Autodesk Fusion 360 part; units mm, degrees
(part 6 of 6)
sketch "Button Layout" plane through (0, 0, 6) normal (0, 0, 1) x (-1, 0, 0)
  line L0 (0, -86.085) -> (0, 0)
  line L1 (0, 0) -> (-270, 0)
  line L2 (-270, 0) -> (-270, -86.085)
  line L3 (-270, -86.085) -> (0, -86.085)
  circle A0 centre (-90, -43) radius 15
  circle A1 centre (-140, -43) radius 15
  circle A2 centre (-40, -43) radius 15
  dimension "d12" = 30
  dimension "d13" = 30
  dimension "d14" = 30
  dimension "d17" = 40
  dimension "d20" = 50
  dimension "d21" = 43
  dimension "d22" = 43
  dimension "d23" = 43
  dimension "d24" = 50
  measures "d12" diameter of A0
  measures "d13" diameter of A1
  measures "d14" diameter of A2
  measures "d17" distance of L0 A2.centre
  measures "d20" distance of A0.centre A1.centre
  measures "d21" distance of L1 A2.centre
  measures "d22" distance of L1 A0.centre
  measures "d23" distance of L1 A1.centre
  measures "d24" distance of A0.centre A2.centre
extrude "Extrude2" cut sketch "Button Layout" against normal blind 6 contours A0 | A1
extrude "Extrude3" cut sketch "Button Layout" against normal blind 6 contours A2
equation "MDFThickness = 6 mm"
equation "d2 = MDFThickness"
equation "controlPanelTopLength = 75 mm"
equation "controlPanelTopWidth = 250 mm"
equation "arcadeButtonDiameter = 30 mm"
equation "d12 = arcadeButtonDiameter"
equation "d13 = arcadeButtonDiameter"
equation "d14 = arcadeButtonDiameter"
equation "d21 = ( 86 / 2 ) * 1 mm"
equation "d22 = ( 86 / 2 ) * 1 mm"
equation "d23 = ( 86 / 2 ) * 1 mm"

design "Sorted Smarties Cover Connector Base"
Autodesk Fusion 360 part; units mm, degrees
sketch "Sorted Smarties Cover Connector Base" plane through (0, 0, 0) normal (0, 0, 1) x (1, 0, 0)
  line L0 (0, 0) -> (30, 0)
  line L1 (30, 0) -> (30, 15)
  line L2 (30, 15) -> (0, 15)
  line L3 (0, 15) -> (0, 0)
  dimension "d5" = 15
  dimension "d6" = 30
  constraint horizontal L0
  constraint vertical L1
  constraint horizontal L2
  constraint vertical L3
  constraint coincident L0.start L3.end
  measures "d5" distance of L0.start L2.end
  measures "d6" distance of L0.start L0.end
extrude "Extrude1" add sketch "Sorted Smarties Cover Connector Base" along normal blind 15
sketch "Connecting Section" plane through (0, 0, 15) normal (0, 0, 1) x (-1, 0, 0)
  line L0 (0, -15) -> (0, 0)
  line L1 (0, 0) -> (-30, 0)
  line L2 (-30, 0) -> (-30, -15)
  line L3 (-30, -15) -> (0, -15)
  line L4 (-30, -11) -> (-4, -11)
  line L5 (-4, -11) -> (-4, -4)
  line L6 (-4, -4) -> (-30, -4)
  line L7 (-30, -4) -> (-30, -11)
  dimension "d7" = 7
  dimension "d8" = 4
  dimension "d9" = 4
  dimension "d10" = 4
  constraint horizontal L4
  constraint vertical L5
  constraint horizontal L6
  constraint vertical L7
  constraint coincident L2 L4.start
  measures "d7" distance of L4 L6
  measures "d8" distance of L1 L6
  measures "d9" distance of L3 L4
  measures "d10" distance of L0 L5
extrude "Extrude2" cut sketch "Connecting Section" against normal blind 11 contours L2 L4 L5 L6 L7
equation "d8 = ( ( 15 - 7 ) / 2 ) * 1 mm"

design "Top Panel"
Autodesk Fusion 360 part; units mm, degrees
sketch "Top Panel" plane through (0, 0, 0) normal (1, 0, 0) x (0, 1, 0)
  line L0 (-0.0158, 146.1836) -> (175.2958, 74.2831)
  line L1 (175.2958, 80.7681) -> (-0.0158, 152.6686)
  line L2 (-0.0158, 152.6686) -> (-0.0158, 146.1836)
  line L3 (175.2958, 80.7681) -> (175.2958, 74.2831)
  dimension "d12" = 189.483
  dimension "d13" = 189.483
  dimension "d14" = 6
  dimension "d18" = 67.7
  constraint vertical L2
  constraint parallel L2 L3
  measures "d12" distance of L1.start L1.end
  measures "d13" distance of L0.start L0.end
  measures "d14" distance of L0 L1
  measures "d18" angle of L0 L3
extrude "Extrude2" add sketch "Top Panel" along normal blind 270
equation "MDFThickness = 6 mm"
equation "topPlateWidth = 210 mm"
equation "baseBreadth = 250 mm"
equation "filletRadius = 8 mm"

design "Lower Wire Management Conduit"
Autodesk Fusion 360 part; units mm, degrees
sketch "16 mm x 16 mm conduit piping shape" plane through (0, 0, 0) normal (1, 0, 0) x (0, 1, 0)
  line L0 (0, 0) -> (16, 0)
  line L1 (16, 0) -> (16, 10)
  line L2 (16, 10) -> (14, 13.9)
  line L3 (14, 13.9) -> (13.1102, 13.4437)
  line L4 (13.1102, 13.4437) -> (15, 9.7585)
  line L5 (15, 9.7585) -> (15, 1)
  line L6 (15, 1) -> (1, 1)
  line L7 (1, 1) -> (1, 9.7585)
  line L8 (1, 9.7585) -> (2.8898, 13.4437)
  line L9 (2.8898, 13.4437) -> (2, 13.9)
  line L10 (2, 13.9) -> (0, 10)
  line L11 (0, 10) -> (0, 0)
  line L12 (0, 16) -> (16, 16)
  line L13 (0, 16) -> (0, 12)
  line L14 (0, 12) -> (1, 12)
  line L15 (1, 12) -> (1, 15)
  line L16 (1, 15) -> (15, 15)
  line L17 (15, 15) -> (15, 12)
  line L18 (15, 12) -> (16, 12)
  line L19 (16, 12) -> (16, 16)
  dimension "d1" = 1
  dimension "d2" = 16
  dimension "d3" = 1
  dimension "d4" = 1
  dimension "d7" = 10
  dimension "d8" = 10
  dimension "d9" = 16
  dimension "d10" = 1
  dimension "d11" = 1
  dimension "d12" = 1
  dimension "d13" = 4
  dimension "d14" = 4
  dimension "d15" = 16
  dimension "d16" = 2
  dimension "d17" = 2
  dimension "d18" = 1
  dimension "d19" = 1
  constraint coincident L0.start L11.end
  constraint horizontal L0
  constraint perpendicular L0 L1
  constraint perpendicular L2 L3
  constraint parallel L1 L5
  constraint perpendicular L5 L6
  constraint perpendicular L6 L7
  constraint perpendicular L0 L11
  constraint horizontal L12
  constraint perpendicular L12 L13
  constraint perpendicular L13 L14
  constraint perpendicular L14 L15
  constraint perpendicular L15 L16
  constraint perpendicular L16 L17
  constraint perpendicular L17 L18
  constraint perpendicular L12 L19
  constraint parallel L8 L10
  constraint parallel L2 L4
  constraint perpendicular L9 L10
  measures "d1" distance of L0 L6
  measures "d2" distance of L1 L11
  measures "d3" distance of L7 L11
  measures "d4" distance of L1 L5
  measures "d7" distance of L0.end L1.end
  measures "d8" distance of L10.end L0.start
  measures "d9" distance of L0 L12
  measures "d10" distance of L12 L16
  measures "d11" distance of L17 L19
  measures "d12" distance of L13 L15
  measures "d13" distance of L12.end L18.end
  measures "d14" distance of L12.start L13.end
  measures "d15" distance of L12.start L12.end
  measures "d16" distance of L1.end L2.end
  measures "d17" distance of L9.end L10.end
  measures "d18" distance of L2.end L3.end
  measures "d19" distance of L8.end L9.end
extrude "Extrude1" add sketch "16 mm x 16 mm conduit piping shape" along normal blind 182 makes body 1 at (60.6667, 5.3333, 16) makes body 2 at (60.6667, 5.3333, 0)
fillet "Fillet1" radius 0.3 18 edges at (91, 0, 16) (91, 16, 16) (91, 16, 12) (91, 0, 12) (91, 1, 12) (91, 15, 12) (91, 1, 15) (91, 15, 15) (91, 0, 10) (91, 16, 10) (91, 14, 13.9) (91, 13.1102, 13.4437) (91, 2, 13.9) (91, 2.8898, 13.4437) (91, 15, 1) (91, 1, 1) (91, 1, 9.7585) (91, 15, 9.7585) on bodies 1 2
equation "d1 = conduitThickness"
equation "d2 = conduitWidth"
equation "d3 = conduitThickness"
equation "d4 = conduitThickness"
equation "conduitThickness = 1 mm"
equation "conduitWidth = 16 mm"
equation "d9 = conduitWidth"
equation "d10 = conduitThickness"
equation "d11 = conduitThickness"
equation "d12 = conduitThickness"
equation "d20 = ( 234 mm ) - ( 2 * ( 26 ) ) * 1 mm"

design "Sorted Smarties Top Support Right"
Autodesk Fusion 360 part; units mm, degrees
sketch "Back Panel Support Left " plane through (0, 0, 0) normal (1, 0, 0) x (0, 1, 0)
  line L0 (0, 0) -> (28, 0)
  line L1 (28, 0) -> (28, 21)
  line L2 (28, 21) -> (0, 21)
  line L3 (0, 21) -> (0, 0)
  dimension "d1" = 21
  dimension "d2" = 28
  constraint horizontal L0
  constraint vertical L1
  constraint horizontal L2
  constraint vertical L3
  constraint coincident L0.start L3.end
  measures "d1" distance of L0.end L1.end
  measures "d2" distance of L0.start L0.end
extrude "Extrude1" add sketch "Back Panel Support Left " along normal blind 21
equation "d2 = 94 mm - 66 mm"

design "Right Side Panel"
Autodesk Fusion 360 part; units mm, degrees
sketch "Side Panel" plane through (0, 0, 0) normal (1, 0, 0) x (0, 1, 0)
  line L0 (0, 0) -> (195, 0)
  line L1 (195, 0) -> (195, 520)
  line L2 (195, 520) -> (-0.3488, 600)
  line L3 (-0.3488, 600) -> (-0.3488, 510)
  line L4 (-0.3488, 510) -> (90, 473)
  line L5 (90, 473) -> (25, 345)
  line L6 (25, 345) -> (-65, 345)
  line L7 (-65, 345) -> (-65, 270)
  line L8 (-65, 270) -> (0, 270)
  line L9 (0, 270) -> (0, 0)
  dimension "d7" = 600
  dimension "d10" = 195
  dimension "d12" = 520
  dimension "d14" = 90
  dimension "d16" = 105
  dimension "d18" = 270
  dimension "d20" = 75
  dimension "d22" = 37
  dimension "d27" = 260
  dimension "d28" = 90
  dimension "d31" = 345
  constraint coincident L0.start L9.end
  constraint horizontal L0
  constraint perpendicular L0 L1
  constraint parallel L1 L3
  constraint parallel L2 L4
  constraint parallel L3 L7
  constraint perpendicular L7 L8
  constraint perpendicular L0 L9
  measures "d7" distance of L0 L2.end
  measures "d10" distance of L0.start L0.end
  measures "d12" distance of L0.end L1.end
  measures "d14" distance of L2.end L3.end
  measures "d16" distance of L1 L4.end
  measures "d18" distance of L8.end L0.start
  measures "d20" distance of L6.end L7.end
  measures "d22" distance of L3.end L4.end
  measures "d27" distance of L1 L7
  measures "d28" distance of L5.end L6.end
  measures "d31" distance of L0.start L5.end
extrude "Extrude1" add sketch "Side Panel" along normal blind 6 makes body 1
fillet "Fillet1" radius 8 10 edges at (3, -65, 345) (3, 25, 345) (3, 90, 473) (3, -0.3488, 510) (3, -0.3488, 600) (3, 195, 520) (3, -65, 270) (3, 0, 270) (3, 0, 0) (3, 195, 0) on bodies 1
sketch "Paint border" plane through (6, 0, 0) normal (1, 0, 0) x (0, 1, 0)
  arc A0 (187, 0) -> (195, 8) centre (187, 8) ccw
  line L0 (195, 8) -> (195, 514.6313)
  arc A1 (195, 514.6313) -> (190.0318, 522.0346) centre (187, 514.6313) ccw
  line L1 (190.0318, 522.0346) -> (10.683, 595.4822)
  arc A2 (10.683, 595.4822) -> (-0.3488, 588.079) centre (7.6512, 588.079) ccw
  line L2 (-0.3488, 588.079) -> (-0.3488, 515.3687)
  arc A3 (-0.3488, 515.3687) -> (4.6194, 507.9654) centre (7.6512, 515.3687) ccw
  line L3 (4.6194, 507.9654) -> (81.9699, 476.2885)
  arc A4 (86.0711, 465.263) -> (81.9699, 476.2885) centre (78.9381, 468.8853) ccw
  line L4 (86.0711, 465.263) -> (27.2231, 349.3778)
  arc A5 (20.0901, 345) -> (27.2231, 349.3778) centre (20.0901, 353) ccw
  line L5 (20.0901, 345) -> (-57, 345)
  arc A6 (-57, 345) -> (-65, 337) centre (-57, 337) ccw
  line L6 (-65, 337) -> (-65, 278)
  arc A7 (-65, 278) -> (-57, 270) centre (-57, 278) ccw
  line L7 (-57, 270) -> (-8, 270)
  arc A8 (0, 262) -> (-8, 270) centre (-8, 262) ccw
  line L8 (0, 262) -> (0, 8)
  arc A9 (0, 8) -> (8, 0) centre (8, 8) ccw
  line L9 (8, 0) -> (187, 0)
  line L10 (10, 6) -> (185, 6)
  line L11 (10, 6) -> (10, 280)
  line L12 (10, 280) -> (-55, 280)
  line L13 (-55, 280) -> (-55, 335)
  line L14 (-55, 335) -> (31.1374, 335)
  line L15 (9.6512, 516.7108) -> (103.8274, 478.1434)
  line L16 (31.1374, 335) -> (103.8274, 478.1434)
  line L17 (187.0159, 512.4636) -> (185, 6)
  line L18 (9.6512, 585.0987) -> (187.0159, 512.4636)
  line L19 (9.6512, 585.0987) -> (9.6512, 516.7108)
  dimension "d32" = 6
  dimension "d33" = 10
  dimension "d34" = 10
  dimension "d35" = 10
  dimension "d36" = 10
  dimension "d37" = 10
  dimension "d41" = 10
  dimension "d42" = 10
  dimension "d43" = 10
  dimension "d44" = 10
  constraint perpendicular L8 L10
  constraint perpendicular L10 L11
  constraint perpendicular L11 L12
  constraint perpendicular L12 L13
  constraint perpendicular L13 L14
  constraint parallel L3 L15
  constraint parallel L4 L16
  measures "d32" distance of L9 L10
  measures "d33" distance of L0 L10.end
  measures "d34" distance of L8 L10.start
  measures "d35" distance of L7 L11.end
  measures "d36" distance of L6 L12.end
  measures "d37" distance of L5 L13.end
  measures "d41" distance of L3 L15
  measures "d42" distance of L4 L16
  measures "d43" distance of L1 L18
  measures "d44" distance of L2 L19
extrude "Extrude2" cut sketch "Paint border" against normal blind 0.1 bodies 1
mirror "Mirror1" about plane through (0, 0, 0) normal (1, 0, 0) of bodies 1 makes body 2
hidden bodies 1
equation "MDFThickness = 6 mm"
equation "filletRadius = 8 mm"
equation "d3 = MDFThickness"
equation "d6 = filletRadius"
equation "d7 = totaHeight"
equation "totaHeight = 600 mm"
equation "baseWidth = 195 mm"
equation "d10 = baseWidth"
equation "backHight = 520 mm"
equation "d12 = backHight"
equation "namePanelHeight = 90 mm"
equation "d14 = namePanelHeight"
equation "neckWidth = 105 mm"
equation "d16 = neckWidth"
equation "bottomFrontHeight = 270 mm"
equation "d18 = bottomFrontHeight"
equation "controlPanelHeight = 75 mm"
equation "d20 = controlPanelHeight"
equation "namePanelFrontDipHeight = 37 mm"
equation "d22 = namePanelFrontDipHeight"
equation "controlPanelTopWidth = 90 mm"
equation "controlPanelTotalWidth = 260 mm"
equation "d27 = controlPanelTotalWidth"
equation "d28 = controlPanelTopWidth"
equation "d31 = bottomFrontHeight + controlPanelHeight"

design "Name Sign Bottom Panel"
Autodesk Fusion 360 part; units mm, degrees
sketch "Name Sign Bottom Panel" plane through (0, 0, 0) normal (1, 0, 0) x (0, 1, 0) in component "Name Sign Bottom Panel"
  line L0 (-0.0158, 146.1836) -> (94.3556, 107.4791)
  line L1 (94.3556, 113.9641) -> (-0.0158, 152.6686)
  line L2 (-0.0158, 152.6686) -> (-0.0158, 146.1836)
  line L3 (94.3556, 113.9641) -> (94.3556, 107.4791)
  dimension "d13" = 102
  dimension "d14" = 6
  dimension "d18" = 67.7
  constraint vertical L2
  constraint parallel L2 L3
  measures "d13" distance of L0.start L0.end
  measures "d14" distance of L0 L1
  measures "d18" angle of L0 L3
extrude "Extrude2" add sketch "Name Sign Bottom Panel" along normal blind 270 in component "Name Sign Bottom Panel"
component "Name Sign Bottom Panel" placed x (1, 0, 0) y (0, 1, 0) z (0, 0, 1) at (0, 0, 0)
equation "MDFThickness = 6 mm"
equation "d14 = MDFThickness"

design "Base Plate"
Autodesk Fusion 360 part; units mm, degrees
sketch "Base Plate" plane through (0, 0, 0) normal (0, 0, 1) x (1, 0, 0)
  line L0 (0, 0) -> (270, 0)
  line L1 (270, 0) -> (270, 175)
  line L2 (270, 175) -> (0, 175)
  line L3 (0, 175) -> (0, 0)
  dimension "d6" = 270
  dimension "d9" = 175
  constraint horizontal L0
  constraint vertical L1
  constraint horizontal L2
  constraint vertical L3
  constraint coincident L0.start L3.end
  measures "d6" distance of L0.start L0.end
  measures "d9" distance of L0.end L1.end
extrude "Extrude1" add sketch "Base Plate" along normal blind 6
equation "MDFThickness = 6 mm"
equation "d2 = MDFThickness"
equation "d9 = sidePanelDepth - 2 * clearance"
equation "clearance = 10 mm"
equation "sidePanelDepth = 195 mm"

design "Back Panel Support Left"
Autodesk Fusion 360 part; units mm, degrees
sketch "Back Panel Support Left " plane through (0, 0, 0) normal (1, 0, 0) x (0, 1, 0)
  line L0 (0, 0) -> (21, 0)
  line L1 (21, 0) -> (21, 478.576)
  line L2 (21, 478.576) -> (0, 478.576)
  line L3 (0, 478.576) -> (0, 0)
  dimension "d1" = 478.576
  dimension "d2" = 21
  constraint horizontal L0
  constraint vertical L1
  constraint horizontal L2
  constraint vertical L3
  constraint coincident L0.start L3.end
  measures "d1" distance of L0.end L1.end
  measures "d2" distance of L0.start L0.end
extrude "Extrude1" add sketch "Back Panel Support Left " along normal blind 21

design "Control Panel Bottom"
Autodesk Fusion 360 part; units mm, degrees
sketch "Control Panel Bottom" plane through (0, 0, 0) normal (0, 0, 1) x (1, 0, 0)
  line L0 (0, 0) -> (270, 0)
  line L1 (270, 0) -> (270, 65)
  line L2 (270, 65) -> (0, 65)
  line L3 (0, 65) -> (0, 0)
  dimension "d5" = 65
  dimension "d7" = 270
  constraint horizontal L0
  constraint vertical L1
  constraint horizontal L2
  constraint vertical L3
  constraint coincident L0.start L3.end
  measures "d5" distance of L0.end L1.end
  measures "d7" distance of L0.start L0.end
extrude "Extrude1" add sketch "Control Panel Bottom" along normal blind 6
equation "MDFThickness = 6 mm"
equation "d2 = MDFThickness"
equation "d5 = sidePanelControlPanelDepth"
equation "sidePanelControlPanelDepth = 65 mm"

design "LED Strip"
Autodesk Fusion 360 part; units mm, degrees
sketch "strip" plane through (0, 0, 0) normal (0, 0, 1) x (1, 0, 0)
  line L0 (0, 0) -> (50, 0)
  line L1 (50, 0) -> (50, 8)
  line L2 (50, 8) -> (0, 8)
  line L3 (0, 8) -> (0, 0)
  dimension "d1" = 50
  dimension "d2" = 8
  constraint horizontal L0
  constraint vertical L1
  constraint horizontal L2
  constraint vertical L3
  constraint coincident L0.start L3.end
  measures "d1" distance of L0.start L0.end
  measures "d2" distance of L0.end L1.end
extrude "Extrude1" add sketch "strip" along normal blind 0.1 makes body 1
sketch "leds" plane through (0, 0, 0.1) normal (0, 0, 1) x (-1, 0, 0)
  line L0 (0, -8) -> (0, 0)
  line L1 (0, 0) -> (-50, 0)
  line L2 (-50, 0) -> (-50, -8)
  line L3 (-50, -8) -> (0, -8)
  line L4 (-5, -5) -> (-8, -5)
  line L5 (-8, -5) -> (-8, -3)
  line L6 (-8, -3) -> (-5, -3)
  line L7 (-5, -3) -> (-5, -5)
  line L8 (-23, -5) -> (-26, -5)
  line L9 (-26, -5) -> (-26, -3)
  line L10 (-26, -3) -> (-23, -3)
  line L11 (-23, -3) -> (-23, -5)
  line L12 (-42, -5) -> (-45, -5)
  line L13 (-45, -5) -> (-45, -3)
  line L14 (-45, -3) -> (-42, -3)
  line L15 (-42, -3) -> (-42, -5)
  dimension "d6" = 5
  dimension "d7" = 15
  dimension "d8" = 3
  dimension "d9" = 3
  dimension "d10" = 3
  dimension "d11" = 5
  dimension "d12" = 16
  dimension "d13" = 2
  dimension "d14" = 2
  dimension "d15" = 2
  dimension "d16" = 3
  constraint horizontal L4
  constraint vertical L5
  constraint horizontal L6
  constraint vertical L7
  constraint horizontal L8
  constraint vertical L9
  constraint horizontal L10
  constraint vertical L11
  constraint horizontal L12
  constraint vertical L13
  constraint horizontal L14
  constraint vertical L15
  constraint collinear L4 L8
  measures "d6" distance of L0 L7
  measures "d7" distance of L5 L11
  measures "d8" distance of L5.end L6.end
  measures "d9" distance of L9.end L10.end
  measures "d10" distance of L13.end L14.end
  measures "d11" distance of L2 L13
  measures "d12" distance of L9 L15
  measures "d13" distance of L4.start L6.end
  measures "d14" distance of L8.start L10.end
  measures "d15" distance of L12.start L14.end
  measures "d16" distance of L3 L4
extrude "Extrude2" add sketch "leds" along normal blind 1 separate body contours L4 L5 L6 L7 | L8 L9 L10 L11 | L12 L13 L14 L15 makes body 2 at (6, 4.3333, 0.1) makes body 3 at (24, 4.3333, 0.1) makes body 4 at (43, 4.3333, 0.1)
sketch "Sketch3" plane through (0, 0, 0.1) normal (0, 0, 1) x (-1, 0, 0)
  line L0 (0, -8) -> (0, 0)
  line L1 (0, 0) -> (-50, 0)
  line L2 (-50, 0) -> (-50, -8)
  line L3 (-50, -8) -> (0, -8)
  circle A0 centre (0, -6) radius 1.5
  circle A1 centre (0, -2) radius 1.5
  circle A2 centre (-50, -6) radius 1.5
  circle A3 centre (-50, -2) radius 1.5
  dimension "d19" = 3
  dimension "d20" = 3
  dimension "d21" = 3
  dimension "d22" = 3
  dimension "d23" = 2
  dimension "d24" = 2
  dimension "d25" = 2
  dimension "d26" = 2
  constraint coincident L2 A2.centre
  constraint coincident L2 A3.centre
  measures "d19" diameter of A2
  measures "d20" diameter of A3
  measures "d21" diameter of A0
  measures "d22" diameter of A1
  measures "d23" distance of L3 A2.centre
  measures "d24" distance of L1 A3.centre
  measures "d25" distance of L3 A0.centre
  measures "d26" distance of L1 A1.centre
extrude "Extrude3" add sketch "Sketch3" along normal blind 0.1 separate body contours L0 A0 | L2 A2 | L0 A1 | L2 A3 picked at (-0.4654, -6.1827) picked at (-49.0815, -5.6726) picked at (-0.2169, -2.4505) picked at (-49.0815, -1.6726) makes body 5 at (0.4654, 6.1827, 0.1) makes body 6 at (49.1724, 2.4778, 0.2) makes body 7 at (0.2169, 2.4505, 0.1) makes body 8 at (49.2956, 5.6062, 0.1)

design "Sorted Smarties Top Panel"
Autodesk Fusion 360 part; units mm, degrees
sketch "Sorted Smarties Top" plane through (0, 0, 0) normal (0, 0, 1) x (1, 0, 0)
  line L0 (0, 0) -> (-270, 0)
  line L1 (-270, 0) -> (-270, 94)
  line L2 (-270, 94) -> (0, 94)
  line L3 (0, 94) -> (0, 0)
  dimension "d2" = 270
  dimension "d3" = 94
  constraint horizontal L0
  constraint vertical L1
  constraint horizontal L2
  constraint vertical L3
  constraint coincident L0.start L3.end
  measures "d2" distance of L0.start L0.end
  measures "d3" distance of L0.start L2.end
extrude "Extrude1" add sketch "Sorted Smarties Top" along normal blind 6
sketch "Sketch2" plane through (0, 0, 0) normal (0, 0, -1) x (1, 0, 0)
  line L0 (-270, -94) -> (0, -94)
  line L1 (0, -94) -> (0, 0)
  line L2 (0, 0) -> (-270, 0)
  line L3 (-270, 0) -> (-270, -94)
  line L4 (-5, -10) -> (-265, -10)
  line L5 (-265, -10) -> (-265, -20)
  line L6 (-265, -20) -> (-5, -20)
  line L7 (-5, -20) -> (-5, -10)
  line L8 (-5, -45) -> (-265, -45)
  line L9 (-265, -45) -> (-265, -55)
  line L10 (-265, -55) -> (-5, -55)
  line L11 (-5, -55) -> (-5, -45)
  dimension "d6" = 10
  dimension "d7" = 10
  dimension "d8" = 10
  dimension "d9" = 25
  dimension "d10" = 5
  dimension "d11" = 5
  dimension "d12" = 5
  dimension "d13" = 5
  constraint horizontal L4
  constraint vertical L5
  constraint horizontal L6
  constraint vertical L7
  constraint horizontal L8
  constraint vertical L9
  constraint horizontal L10
  constraint vertical L11
  measures "d6" distance of L2 L4
  measures "d7" distance of L4.start L6.end
  measures "d8" distance of L8.start L10.end
  measures "d9" distance of L6 L8
  measures "d10" distance of L3 L5
  measures "d11" distance of L1 L7
  measures "d12" distance of L1 L11
  measures "d13" distance of L3 L9
extrude "Extrude2" cut sketch "Sketch2" against normal blind 4 contours L4 L5 L6 L7 | L8 L9 L10 L11
sketch "Sketch3" plane through (0, 0, 4) normal (0, 0, -1) x (1, 0, 0)
  line L0 (-5, -20) -> (-5, -10)
  line L1 (-5, -10) -> (-265, -10)
  line L2 (-265, -10) -> (-265, -20)
  line L3 (-265, -20) -> (-5, -20)
  line L4 (-5, -10) -> (-15, -10)
  line L5 (-15, -10) -> (-15, -20)
  line L6 (-15, -20) -> (-5, -20)
  line L7 (-5, -20) -> (-5, -10)
  line L8 (-5, -45) -> (-15, -45)
  line L9 (-15, -45) -> (-15, -55)
  line L10 (-15, -55) -> (-5, -55)
  line L11 (-5, -55) -> (-5, -45)
  constraint horizontal L4
  constraint vertical L5
  constraint horizontal L6
  constraint vertical L7
  constraint coincident L3 L5.end
  constraint coincident L0.end L1.start
  constraint horizontal L8
  constraint vertical L9
  constraint horizontal L10
  constraint vertical L11
extrude "Extrude3" cut sketch "Sketch3" against normal blind 2 contours L0 L1 L3 L4 L5 L6 L7 | L8 L9 L10 L11
equation "MDFThickness = 6 mm"
equation "d3 = 100 mm - MDFThickness"
equation "d4 = MDFThickness"

design "Name Sign Support Right"
Autodesk Fusion 360 part; units mm, degrees
sketch "Name Sign Support" plane through (0, 0, 0) normal (1, 0, 0) x (0, 1, 0) in component "Name Sign Support (1)"
  line L0 (-0.0158, 97.2466) -> (23.9842, 87.4035)
  line L1 (23.9842, 142.8255) -> (-0.0158, 152.6686)
  line L2 (-0.0158, 152.6686) -> (-0.0158, 97.2466)
  line L3 (23.9842, 142.8255) -> (23.9842, 87.4035)
  dimension "d18" = 67.7
  dimension "d8" = 24
  dimension "d9" = 55.422
  constraint vertical L2
  constraint parallel L2 L3
  measures "d18" angle of L0 L3
  measures "d8" distance of L2 L3
  measures "d9" distance of L1.end L0.start
extrude "Extrude2" add sketch "Name Sign Support" along normal blind 12 in component "Name Sign Support (1)"
component "Name Sign Support Right" placed x (1, 0, 0) y (0, 1, 0) z (0, 0, 1) at (0, 0, 0)
component "Name Sign Support (1)" placed x (1, 0, 0) y (0, 1, 0) z (0, 0, 1) at (0, 0, 0) in component "Name Sign Support Right"
equation "d19 = pineThickness"
equation "pineThickness = 12 mm"

design "Colour Detection Mechanism Conduit"
Autodesk Fusion 360 part; units mm, degrees
sketch "16 mm x 16 mm conduit piping shape" plane through (0, 0, 0) normal (1, 0, 0) x (0, 1, 0)
  line L0 (0, 0) -> (16, 0)
  line L1 (16, 0) -> (16, 10)
  line L2 (16, 10) -> (14, 13.9)
  line L3 (14, 13.9) -> (13.1102, 13.4437)
  line L4 (13.1102, 13.4437) -> (15, 9.7585)
  line L5 (15, 9.7585) -> (15, 1)
  line L6 (15, 1) -> (1, 1)
  line L7 (1, 1) -> (1, 9.7585)
  line L8 (1, 9.7585) -> (2.8898, 13.4437)
  line L9 (2.8898, 13.4437) -> (2, 13.9)
  line L10 (2, 13.9) -> (0, 10)
  line L11 (0, 10) -> (0, 0)
  line L12 (0, 16) -> (16, 16)
  line L13 (0, 16) -> (0, 12)
  line L14 (0, 12) -> (1, 12)
  line L15 (1, 12) -> (1, 15)
  line L16 (1, 15) -> (15, 15)
  line L17 (15, 15) -> (15, 12)
  line L18 (15, 12) -> (16, 12)
  line L19 (16, 12) -> (16, 16)
  dimension "d1" = 1
  dimension "d2" = 16
  dimension "d3" = 1
  dimension "d4" = 1
  dimension "d7" = 10
  dimension "d8" = 10
  dimension "d9" = 16
  dimension "d10" = 1
  dimension "d11" = 1
  dimension "d12" = 1
  dimension "d13" = 4
  dimension "d14" = 4
  dimension "d15" = 16
  dimension "d16" = 2
  dimension "d17" = 2
  dimension "d18" = 1
  dimension "d19" = 1
  constraint coincident L0.start L11.end
  constraint horizontal L0
  constraint perpendicular L0 L1
  constraint perpendicular L2 L3
  constraint parallel L1 L5
  constraint perpendicular L5 L6
  constraint perpendicular L6 L7
  constraint perpendicular L0 L11
  constraint horizontal L12
  constraint perpendicular L12 L13
  constraint perpendicular L13 L14
  constraint perpendicular L14 L15
  constraint perpendicular L15 L16
  constraint perpendicular L16 L17
  constraint perpendicular L17 L18
  constraint perpendicular L12 L19
  constraint parallel L8 L10
  constraint parallel L2 L4
  constraint perpendicular L9 L10
  measures "d1" distance of L0 L6
  measures "d2" distance of L1 L11
  measures "d3" distance of L7 L11
  measures "d4" distance of L1 L5
  measures "d7" distance of L0.end L1.end
  measures "d8" distance of L10.end L0.start
  measures "d9" distance of L0 L12
  measures "d10" distance of L12 L16
  measures "d11" distance of L17 L19
  measures "d12" distance of L13 L15
  measures "d13" distance of L12.end L18.end
  measures "d14" distance of L12.start L13.end
  measures "d15" distance of L12.start L12.end
  measures "d16" distance of L1.end L2.end
  measures "d17" distance of L9.end L10.end
  measures "d18" distance of L2.end L3.end
  measures "d19" distance of L8.end L9.end
extrude "Extrude1" add sketch "16 mm x 16 mm conduit piping shape" along normal blind 94 makes body 1 at (31.3333, 5.3333, 16) makes body 2 at (31.3333, 5.3333, 0)
fillet "Fillet1" radius 0.3 18 edges at (47, 0, 16) (47, 16, 16) (47, 16, 12) (47, 0, 12) (47, 1, 12) (47, 15, 12) (47, 1, 15) (47, 15, 15) (47, 0, 10) (47, 16, 10) (47, 14, 13.9) (47, 13.1102, 13.4437) (47, 2, 13.9) (47, 2.8898, 13.4437) (47, 15, 1) (47, 1, 1) (47, 1, 9.7585) (47, 15, 9.7585) on bodies 1 2
sketch "Sketch2" plane through (0, 0, 0) normal (0, -1, 0) x (1, 0, 0)
  line L0 (94, 9.9276) -> (0, 9.9276)
  line L1 (0, 9.9276) -> (0, 0)
  line L2 (0, 0) -> (94, 0)
  line L3 (94, 0) -> (94, 9.9276)
  line L4 (0, 15) -> (20, 15)
  line L5 (20, 15) -> (20, 1)
  line L6 (20, 1) -> (0, 1)
  line L7 (0, 1) -> (0, 15)
  line L8 (45, 15) -> (55, 15)
  line L9 (55, 15) -> (55, 1)
  line L10 (55, 1) -> (45, 1)
  line L11 (45, 1) -> (45, 15)
  dimension "d25" = 20
  dimension "d26" = 1
  dimension "d27" = 25
  dimension "d28" = 10
  dimension "d29" = 1
  constraint horizontal L4
  constraint vertical L5
  constraint horizontal L6
  constraint vertical L7
  constraint horizontal L8
  constraint vertical L9
  constraint horizontal L10
  constraint vertical L11
  measures "d25" distance of L5 L7
  measures "d26" distance of L2 L6
  measures "d27" distance of L5 L11
  measures "d28" distance of L9.end L10.end
  measures "d29" distance of L2 L10
extrude "Extrude2" cut sketch "Sketch2" against normal blind 3 contours L0 L9 L10 L11 | L0 L8 L9 L11 | L0 L1 L5 L6 L7 | L0 L4 L5 L7 bodies 2
sketch "Sketch3" plane through (0, 16, 0) normal (0, 1, 0) x (-1, 0, 0)
  line L0 (0, 9.9276) -> (-94, 9.9276)
  line L1 (-94, 9.9276) -> (-94, 0)
  line L2 (-94, 0) -> (0, 0)
  line L3 (0, 0) -> (0, 9.9276)
  line L4 (0, 15) -> (-20, 15)
  line L5 (-20, 15) -> (-20, 1)
  line L6 (-20, 1) -> (0, 1)
  line L7 (0, 1) -> (0, 15)
  dimension "d32" = 20
  dimension "d33" = 1
  constraint horizontal L4
  constraint vertical L5
  constraint horizontal L6
  constraint vertical L7
  measures "d32" distance of L4.start L4.end
  measures "d33" distance of L2 L6
extrude "Extrude3" cut sketch "Sketch3" against normal blind 3 contours L0 L3 L5 L6 L7 | L0 L4 L5 L7 bodies 2
sketch "Sketch4" plane through (0, 16, 0) normal (0, 1, 0) x (-1, 0, 0)
  line L0 (-20, 1) -> (-20, 9.9276)
  line L1 (-20, 9.9276) -> (-94, 9.9276)
  line L2 (-94, 9.9276) -> (-94, 0)
  line L3 (-94, 0) -> (0, 0)
  line L4 (0, 0) -> (0, 1)
  line L5 (0, 1) -> (-20, 1)
  line L6 (-45, 1) -> (-45, 15)
  line L7 (-45, 15) -> (-55, 15)
  line L8 (-55, 15) -> (-55, 1)
  line L9 (-55, 1) -> (-45, 1)
  line L10 (-55, 1) -> (-40, 1)
  line L11 (-40, 1) -> (-40, 15)
  line L12 (-40, 15) -> (-55, 15)
  line L13 (-55, 15) -> (-55, 1)
  dimension "d36" = 15
  constraint horizontal L10
  constraint vertical L11
  constraint horizontal L12
  constraint vertical L13
  constraint coincident L8.end L9.start
  constraint collinear L7 L12
  measures "d36" distance of L8.end L10.end
extrude "Extrude4" cut sketch "Sketch4" against normal blind 3 contours L1 L6 L10 L11 | L1 L6 L11 L12 | L1 L6 L8 L9 L10 L13 | L1 L6 L7 L8 L12 L13 bodies 2
equation "d1 = conduitThickness"
equation "d2 = conduitWidth"
equation "d3 = conduitThickness"
equation "d4 = conduitThickness"
equation "conduitThickness = 1 mm"
equation "conduitWidth = 16 mm"
equation "d9 = conduitWidth"
equation "d10 = conduitThickness"
equation "d11 = conduitThickness"
equation "d12 = conduitThickness"
